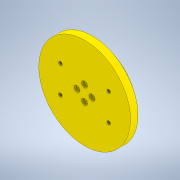
# Autodesk Inventor part: Podstawa2
Saved by Autodesk Inventor 2022 (Build 260153000, 153)
## iProperties
Created: 2023-11-10
Part Number: Podstawa2
Material: Ogólny
Document SubType Name: Modeling
Designer: nosal
Density: 1 g/cm^3
Appearance: Domyślna
Author: nosal
Autodesk Inventor part; units mm, degrees
ref_plane "YZ Plane" through (0, 0, 0) normal (1, 0, 0) x (0, 1, 0)
ref_plane "XZ Plane" through (0, 0, 0) normal (0, 1, 0) x (-1, 0, 0)
ref_plane "XY Plane" through (0, 0, 0) normal (0, 0, 1) x (1, 0, 0)
sketch "Szkic1" plane through (0, 0, 0) normal (0, 0, 1) x (1, 0, 0)
  circle A0 centre (0, 0) radius 10.75
  circle A1 centre (0, 0) radius 11.25
  circle A2 centre (0, 0) radius 43
  dimension "d0" = 21.5
  dimension "d1" = 0.5
  dimension "d2" = 86
  constraints: 3 centre point, 2 coincident
  measures "d0" diameter of A0
  measures "d1" radial gap between concentric circles of A0 A1
  measures "d2" diameter of A2
extrude "Wyciągnięcie proste1" add sketch "Szkic1" along normal blind 10 contours A0 | A1 | A2
sketch "Szkic2" plane through (0, 0, 10) normal (0, 0, 1) x (1, 0, 0)
  circle A0 centre (0, 0) radius 3.5
  point P0 (7.1, 0)
  point P1 (0, 7.1)
  point P2 (-7.1, 0)
  point P3 (0, -7.1)
  dimension "d5" = 7.1
  dimension "d6" = 7.1
  dimension "d7" = 7.1
  dimension "d8" = 7.1
  dimension "d9" = 7
  constraints: 1 centre point, 1 coincident
  measures "d5" distance of point (7.1, 0) point (0, 0)
  measures "d6" distance of point (0, 7.1) point (0, 0)
  measures "d7" distance of point (0, -7.1) point (0, 0)
  measures "d8" distance of point (-7.1, 0) point (0, 0)
  measures "d9" diameter of A0
hole "Otwór1" at (7.1, 0, 10) at (0, 7.1, 10) at (-7.1, 0, 10) at (0, -7.1, 10) direction (0, 0, -1) diameter 1.567 end through all thread size "M2x0.4" designation "M2" class "6H" standard "GB Metric profile"
sketch "Szkic3" plane through (0, 0, 0) normal (0, 0, -1) x (-1, 0, 0)
  circle A0 centre (0, 0) radius 11.5
  dimension "d17" = 23
  constraints: 1 centre point, 1 coincident
  measures "d17" diameter of A0
extrude "Wyciągnięcie proste2" cut sketch "Szkic3" against normal blind 2
sketch "Szkic4" plane through (0, 0, 2) normal (0, 0, -1) x (-1, 0, 0)
  circle A0 centre (0, 0) radius 3.5
  dimension "d20" = 7
  constraints: 1 centre point, 1 coincident
  measures "d20" diameter of A0
extrude "Wyciągnięcie proste3" cut sketch "Szkic4" against normal blind 1
sketch "Szkic5" plane through (0, 0, 10) normal (0, 0, 1) x (1, 0, 0)
  circle A0 centre (-7.1, 0) radius 0.7835 projected
  circle A1 centre (7.1, 0) radius 0.7835 projected
  circle A2 centre (0, 7.1) radius 0.7835 projected
  circle A3 centre (0, -7.1) radius 0.7835 projected
  circle A4 centre (0, 0) radius 43 projected
extrude "Wyciągnięcie proste4" cut sketch "Szkic5" against normal blind 5
sketch "Szkic6" plane through (0, 0, 5) normal (0, 0, 1) x (1, 0, 0)
  circle A0 centre (0, -7.1) radius 0.7835 projected
  circle A1 centre (7.1, 0) radius 0.7835 projected
  circle A2 centre (-7.1, 0) radius 0.7835 projected
  circle A3 centre (0, 7.1) radius 0.7835 projected
  circle A4 centre (0, -7.1) radius 2.75
  circle A5 centre (-7.1, 0) radius 0.7835 projected
  circle A6 centre (-7.1, 0) radius 2.75
  circle A7 centre (0, 7.1) radius 2.75
  circle A8 centre (7.1, 0) radius 0.7835 projected
  circle A9 centre (7.1, 0) radius 2.75
  point P0 (0, 0)
  dimension "d25" = 5.5
  dimension "d26" = 5.5
  dimension "d27" = 5.5
  dimension "d28" = 5.5
  constraints: 4 centre point, 4 coincident
  measures "d25" diameter of A4
  measures "d26" diameter of A6
  measures "d27" diameter of A7
  measures "d28" diameter of A9
extrude "Wyciągnięcie proste5" cut sketch "Szkic6" against normal blind 2 contours A3 | A4 | A6 | A7 | A9
sketch "Szkic9" plane through (0, 0, 0) normal (0, 0, -1) x (-1, 0, 0)
  circle A0 centre (0, 0) radius 11.5 projected
  circle A1 centre (0, 0) radius 43 projected
  circle A2 centre (0, 0) radius 37
  dimension "d36" = 6
  constraints: 1 centre point
  measures "d36" radial gap between concentric circles of A1 A2
extrude "Wyciągnięcie proste7" add sketch "Szkic9" along normal blind 2 contours A1
sketch "Szkic10" plane through (0, 0, -2) normal (0, 0, -1) x (-1, 0, 0)
  circle A0 centre (0, 0) radius 43 projected
  circle A1 centre (0, 0) radius 37 projected
  circle A2 centre (0, 0) radius 39
  dimension "d39" = 2
  constraints: 1 centre point
  measures "d39" radial gap between concentric circles of A1 A2
extrude "Wyciągnięcie proste8" add sketch "Szkic10" along normal blind 3 contours A2
sketch "Szkic12" plane through (0, 0, 5) normal (0, 0, 1) x (1, 0, 0)
  line L0 (-30.65, -20.8055) -> (30.65, -20.8055)
  line L1 (30.65, -20.8055) -> (30.65, 20.8055)
  line L2 (30.65, 20.8055) -> (-30.65, 20.8055)
  line L3 (-30.65, 20.8055) -> (-30.65, -20.8055)
  line L4 (-30.65, -20.8055) -> (30.65, 20.8055) construction
  line L5 (30.65, -20.8055) -> (-30.65, 20.8055) construction
  point P0 (0, 0)
  point P1 (-22.65, 12.8055)
  point P2 (-22.65, -12.8055)
  point P3 (22.65, 12.8055)
  point P4 (22.65, -12.8055)
  dimension "d59" = 61.3
  dimension "d60" = 41.611
  dimension "d61" = 8
  dimension "d62" = 8
  dimension "d63" = 8
  dimension "d64" = 8
  dimension "d65" = 8
  dimension "d66" = 8
  dimension "d67" = 8
  dimension "d68" = 8
  constraints: 12 end point, 2 midpoint, 2 parallel, 1 horizontal, 1 perpendicular
  measures "d59" distance of L1.end L2.end
  measures "d60" distance of L0.end L1.end
  measures "d61" distance from line of L2 point (-22.65, 12.805)
  measures "d62" distance from line of L3 point (-22.65, 12.805)
  measures "d63" distance from line of L2 point (22.65, 12.806)
  measures "d64" distance from line of L0 point (22.65, -12.805)
  measures "d65" distance from line of L0 point (-22.65, -12.805)
  measures "d66" distance from line of L3 point (-22.65, -12.805)
  measures "d67" distance from line of L1 point (22.65, -12.805)
  measures "d68" distance from line of L1 point (22.65, 12.806)
hole "Otwór3" at (-22.65, 12.8055, 5) at (-22.65, -12.8055, 5) at (22.65, 12.8055, 5) at (22.65, -12.8055, 5) direction (0, 0, -1) diameter 3.242 end through all thread size "M4x0.7" designation "M4" class "6H" standard "GB Metric profile"
equation "\"d6\" = d5"
equation "\"d7\" = d6"
equation "\"d8\" = d6"
